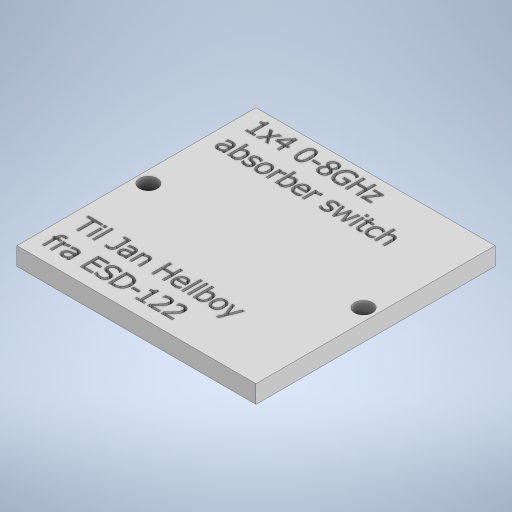
# Autodesk Inventor part: switch cover
Saved by Autodesk Inventor 2023.5 (Build 275446000, 446)
## iProperties
Created: 2025-10-22
Part Number: switch cover
Material: Generic
Document SubType Name: Modeling
Designer: Mikke
Density: 1 g/cm^3
Appearance: Default
Author: Mikke
Autodesk Inventor part; units mm, degrees
(part 1 of 2)
ref_plane "YZ Plane" through (0, 0, 0) normal (1, 0, 0) x (0, 1, 0)
ref_plane "XZ Plane" through (0, 0, 0) normal (0, 1, 0) x (-1, 0, 0)
ref_plane "XY Plane" through (0, 0, 0) normal (0, 0, 1) x (1, 0, 0)
sketch "Sketch1" plane through (0, 0, 0) normal (0, 1, 0) x (-1, 0, 0)
  line L0 (-20, 20) -> (20, 20)
  line L1 (20, 20) -> (20, -20)
  line L2 (20, -20) -> (-20, -20)
  line L3 (-20, -20) -> (-20, 20)
  line L4 (-20, 20) -> (20, -20) construction
  line L5 (20, 20) -> (-20, -20) construction
  line L6 (20, 0) -> (18, 0)
  circle A0 centre (18, 0) radius 1.5
  line L7 (-20, 0) -> (-18, 0)
  circle A1 centre (-18, 0) radius 1.5
  point P0 (0, 0)
  dimension "d0" = 40
  dimension "d1" = 40
  dimension "d2" = 2
  dimension "d3" = 3
  dimension "d4" = 2
  dimension "d5" = 3
  constraints: 16 end point, 4 midpoint, 3 horizontal, 2 centre point, 2 coincident, 2 parallel, 1 perpendicular
  measures "d0" distance of L1.end L2.end
  measures "d1" distance of L0.end L1.end
  measures "d2" distance of L6.start L6.end
  measures "d3" diameter of A0
  measures "d4" distance of L7.start L7.end
  measures "d5" diameter of A1
extrude "Extrusion1" add sketch "Sketch1" along normal blind 3
sketch "Sketch2" plane through (0, 3, 0) normal (0, 1, 0) x (1, 0, 0)
  line L0 (-18.035, 18.8782) -> (18.3992, 18.8782) construction
  line L1 (18.3992, 18.8782) -> (18.3992, 9.0682) construction
  line L2 (18.3992, 9.0682) -> (-18.035, 9.0682) construction
  line L3 (-18.035, 9.0682) -> (-18.035, 18.8782) construction
  line L4 (-18.3377, -9.5579) -> (18.7673, -9.5579) construction
  line L5 (18.7673, -9.5579) -> (18.7673, -19.1286) construction
  line L6 (18.7673, -19.1286) -> (-18.3377, -19.1286) construction
  line L7 (-18.3377, -19.1286) -> (-18.3377, -9.5579) construction
  line L8 (-16.0862, 15.761) -> (-17.5731, 15.761)
  line L9 (-17.5731, 15.761) -> (-17.5731, 16.0722)
  line L10 (-17.5731, 16.0722) -> (-17.0198, 16.0722)
  line L11 (-17.0198, 16.0722) -> (-17.0198, 18.1149)
  line L12 (-17.0198, 18.1149) -> (-17.5731, 18.1149)
  line L13 (-17.5731, 18.1149) -> (-17.5731, 18.394)
  spline S0 degree 2 poles (-17.5731, 18.394) (-17.2594, 18.394) (-16.963, 18.5719) (-16.9433, 18.8189) knots 0 0 0 1 2 2 2
  line L14 (-16.9433, 18.8189) -> (-16.6271, 18.8189)
  line L15 (-16.6271, 18.8189) -> (-16.6271, 16.0722)
  line L16 (-16.6271, 16.0722) -> (-16.0862, 16.0722)
  line L17 (-16.0862, 16.0722) -> (-16.0862, 15.761)
  line L18 (-13.6927, 15.761) -> (-14.1645, 15.761)
  line L19 (-14.1645, 15.761) -> (-14.7203, 16.6206)
  line L20 (-14.7203, 16.6206) -> (-15.2908, 15.761)
  line L21 (-15.2908, 15.761) -> (-15.728, 15.761)
  line L22 (-15.728, 15.761) -> (-14.9352, 16.8947)
  line L23 (-14.9352, 16.8947) -> (-15.7206, 18.0482)
  line L24 (-15.7206, 18.0482) -> (-15.2488, 18.0482)
  line L25 (-15.2488, 18.0482) -> (-14.6956, 17.1961)
  line L26 (-14.6956, 17.1961) -> (-14.1299, 18.0482)
  line L27 (-14.1299, 18.0482) -> (-13.6927, 18.0482)
  line L28 (-13.6927, 18.0482) -> (-14.4807, 16.9194)
  line L29 (-14.4807, 16.9194) -> (-13.6927, 15.761)
  line L30 (-11.4895, 16.8083) -> (-11.8526, 16.8083)
  line L31 (-11.8526, 16.8083) -> (-11.8526, 15.761)
  line L32 (-11.8526, 15.761) -> (-12.2453, 15.761)
  line L33 (-12.2453, 15.761) -> (-12.2453, 16.8083)
  line L34 (-12.2453, 16.8083) -> (-13.5915, 16.8083)
  line L35 (-13.5915, 16.8083) -> (-13.5915, 17.2381)
  line L36 (-13.5915, 17.2381) -> (-12.228, 18.809)
  line L37 (-12.228, 18.809) -> (-11.8526, 18.809)
  line L38 (-11.8526, 18.809) -> (-11.8526, 17.1368)
  line L39 (-11.8526, 17.1368) -> (-11.4895, 17.1368)
  line L40 (-11.4895, 17.1368) -> (-11.4895, 16.8083)
  line L41 (-12.2453, 17.1368) -> (-12.2453, 18.3274)
  line L42 (-12.2453, 18.3274) -> (-13.2704, 17.1368)
  line L43 (-13.2704, 17.1368) -> (-12.2453, 17.1368)
  spline S1 degree 2 poles (-7.9574, 17.285) (-7.9574, 16.465) (-8.4341, 15.6968) (-8.9305, 15.6968) knots 0 0 0 1 2 2 2
  spline S2 degree 2 poles (-8.9305, 15.6968) (-9.4344, 15.6968) (-9.9062, 16.4798) (-9.9062, 17.2825) knots 0 0 0 1 2 2 2
  spline S3 degree 2 poles (-9.9062, 17.2825) (-9.9062, 18.1075) (-9.4295, 18.8708) (-8.9305, 18.8708) knots 0 0 0 1 2 2 2
  spline S4 degree 2 poles (-8.9305, 18.8708) (-8.4291, 18.8708) (-7.9574, 18.0804) (-7.9574, 17.285) knots 0 0 0 1 2 2 2
  spline S5 degree 2 poles (-8.481, 16.3563) (-8.4217, 16.507) (-8.3723, 16.9713) (-8.3723, 17.285) knots 0 0 0 1 2 2 2
  spline S6 degree 2 poles (-8.3723, 17.285) (-8.3723, 17.5987) (-8.4217, 18.0606) (-8.4835, 18.2162) knots 0 0 0 1 2 2 2
  spline S7 degree 2 poles (-8.4835, 18.2162) (-8.5452, 18.3718) (-8.7601, 18.5324) (-8.9305, 18.5324) knots 0 0 0 1 2 2 2
  spline S8 degree 2 poles (-8.9305, 18.5324) (-9.101, 18.5324) (-9.3208, 18.3718) (-9.385, 18.2113) knots 0 0 0 1 2 2 2
  spline S9 degree 2 poles (-9.385, 18.2113) (-9.4468, 18.0557) (-9.4912, 17.5814) (-9.4912, 17.2825) knots 0 0 0 1 2 2 2
  spline S10 degree 2 poles (-9.4912, 17.2825) (-9.4912, 16.9614) (-9.4517, 16.5317) (-9.3875, 16.3637) knots 0 0 0 1 2 2 2
  spline S11 degree 2 poles (-9.3875, 16.3637) (-9.3282, 16.2056) (-9.1084, 16.0352) (-8.9305, 16.0352) knots 0 0 0 1 2 2 2
  spline S12 degree 2 poles (-8.9305, 16.0352) (-8.7626, 16.0352) (-8.5428, 16.1957) (-8.481, 16.3563) knots 0 0 0 1 2 2 2
  line L44 (-6.4506, 16.9096) -> (-7.6041, 16.9096)
  line L45 (-7.6041, 16.9096) -> (-7.6041, 17.2801)
  line L46 (-7.6041, 17.2801) -> (-6.4506, 17.2801)
  line L47 (-6.4506, 17.2801) -> (-6.4506, 16.9096)
  spline S13 degree 2 poles (-5.1243, 15.6918) (-5.3515, 15.6918) (-5.7245, 15.8277) (-5.8554, 15.9537) knots 0 0 0 1 2 2 2
  spline S14 degree 2 poles (-5.8554, 15.9537) (-5.9838, 16.0772) (-6.1172, 16.4131) (-6.1172, 16.6033) knots 0 0 0 1 2 2 2
  spline S15 degree 2 poles (-6.1172, 16.6033) (-6.1172, 16.8503) (-5.8529, 17.2652) (-5.601, 17.3887) knots 0 0 0 1 2 2 2
  line L48 (-5.601, 17.3887) -> (-5.601, 17.4011)
  spline S16 degree 2 poles (-5.601, 17.4011) (-5.8257, 17.532) (-6.0431, 17.8432) (-6.0431, 18.0754) knots 0 0 0 1 2 2 2
  spline S17 degree 2 poles (-6.0431, 18.0754) (-6.0431, 18.4187) (-5.5244, 18.8782) (-5.1243, 18.8782) knots 0 0 0 1 2 2 2
  spline S18 degree 2 poles (-5.1243, 18.8782) (-4.7093, 18.8782) (-4.2079, 18.4434) (-4.2079, 18.1026) knots 0 0 0 1 2 2 2
  spline S19 degree 2 poles (-4.2079, 18.1026) (-4.2079, 17.8976) (-4.4475, 17.4974) (-4.6722, 17.3838) knots 0 0 0 1 2 2 2
  line L49 (-4.6722, 17.3838) -> (-4.6722, 17.3715)
  spline S20 degree 2 poles (-4.6722, 17.3715) (-4.4055, 17.248) (-4.1313, 16.8923) (-4.1313, 16.6107) knots 0 0 0 1 2 2 2
  spline S21 degree 2 poles (-4.1313, 16.6107) (-4.1313, 16.2204) (-4.6994, 15.6918) (-5.1243, 15.6918) knots 0 0 0 1 2 2 2
  spline S22 degree 2 poles (-4.5512, 16.5712) (-4.5512, 16.7589) (-4.6994, 16.9812) (-4.9094, 17.0948) knots 0 0 0 1 2 2 2
  spline S23 degree 2 poles (-4.9094, 17.0948) (-4.9785, 17.1343) (-5.2107, 17.2257) (-5.3564, 17.285) knots 0 0 0 1 2 2 2
  spline S24 degree 2 poles (-5.3564, 17.285) (-5.5244, 17.1739) (-5.7047, 16.8429) (-5.7047, 16.6329) knots 0 0 0 1 2 2 2
  spline S25 degree 2 poles (-5.7047, 16.6329) (-5.7047, 16.3563) (-5.3713, 15.9957) (-5.1193, 15.9957) knots 0 0 0 1 2 2 2
  spline S26 degree 2 poles (-5.1193, 15.9957) (-4.8624, 15.9957) (-4.5512, 16.3044) (-4.5512, 16.5712) knots 0 0 0 1 2 2 2
  spline S27 degree 2 poles (-4.608, 18.0976) (-4.608, 18.3027) (-4.8822, 18.5768) (-5.1267, 18.5768) knots 0 0 0 1 2 2 2
  spline S28 degree 2 poles (-5.1267, 18.5768) (-5.349, 18.5768) (-5.6331, 18.3323) (-5.6331, 18.1223) knots 0 0 0 1 2 2 2
  spline S29 degree 2 poles (-5.6331, 18.1223) (-5.6331, 17.9717) (-5.4873, 17.7617) (-5.3416, 17.6777) knots 0 0 0 1 2 2 2
  spline S30 degree 2 poles (-5.3416, 17.6777) (-5.2799, 17.6432) (-5.018, 17.5221) (-4.9118, 17.4875) knots 0 0 0 1 2 2 2
  spline S31 degree 2 poles (-4.9118, 17.4875) (-4.734, 17.6234) (-4.608, 17.9124) (-4.608, 18.0976) knots 0 0 0 1 2 2 2
  spline S32 degree 2 poles (-2.3949, 15.7017) (-2.7185, 15.7017) (-3.2544, 15.8993) (-3.4471, 16.0994) knots 0 0 0 1 2 2 2
  spline S33 degree 2 poles (-3.4471, 16.0994) (-3.6398, 16.3019) (-3.8448, 16.8997) (-3.8448, 17.2875) knots 0 0 0 1 2 2 2
  spline S34 degree 2 poles (-3.8448, 17.2875) (-3.8448, 17.6555) (-3.6373, 18.2384) (-3.4446, 18.4459) knots 0 0 0 1 2 2 2
  spline S35 degree 2 poles (-3.4446, 18.4459) (-3.2594, 18.646) (-2.716, 18.8633) (-2.3924, 18.8633) knots 0 0 0 1 2 2 2
  spline S36 degree 2 poles (-2.3924, 18.8633) (-2.2368, 18.8633) (-1.9552, 18.8189) (-1.8268, 18.7794) knots 0 0 0 1 2 2 2
  spline S37 degree 2 poles (-1.8268, 18.7794) (-1.723, 18.7497) (-1.4711, 18.641) (-1.3945, 18.6015) knots 0 0 0 1 2 2 2
  line L50 (-1.3945, 18.6015) -> (-1.3945, 18.1125)
  line L51 (-1.3945, 18.1125) -> (-1.4291, 18.1125)
  spline S38 degree 2 poles (-1.4291, 18.1125) (-1.5057, 18.1792) (-1.6662, 18.3002) (-1.8144, 18.3693) knots 0 0 0 1 2 2 2
  spline S39 degree 2 poles (-1.8144, 18.3693) (-1.9379, 18.4311) (-2.2566, 18.5126) (-2.4393, 18.5126) knots 0 0 0 1 2 2 2
  spline S40 degree 2 poles (-2.4393, 18.5126) (-2.879, 18.5126) (-3.4224, 17.8506) (-3.4224, 17.2998) knots 0 0 0 1 2 2 2
  spline S41 degree 2 poles (-3.4224, 17.2998) (-3.4224, 16.9935) (-3.2791, 16.5341) (-3.1433, 16.376) knots 0 0 0 1 2 2 2
  spline S42 degree 2 poles (-3.1433, 16.376) (-3.0124, 16.218) (-2.6419, 16.0525) (-2.4097, 16.0525) knots 0 0 0 1 2 2 2
  spline S43 degree 2 poles (-2.4097, 16.0525) (-2.2393, 16.0525) (-1.8984, 16.1019) (-1.7823, 16.1513) knots 0 0 0 1 2 2 2
  line L52 (-1.7823, 16.1513) -> (-1.7823, 16.9392)
  line L53 (-1.7823, 16.9392) -> (-2.4887, 16.9392)
  line L54 (-2.4887, 16.9392) -> (-2.4887, 17.2949)
  line L55 (-2.4887, 17.2949) -> (-1.3822, 17.2949)
  line L56 (-1.3822, 17.2949) -> (-1.3822, 15.9635)
  spline S44 degree 2 poles (-1.3822, 15.9635) (-1.4587, 15.929) (-1.7206, 15.8228) (-1.8317, 15.7906) knots 0 0 0 1 2 2 2
  spline S45 degree 2 poles (-1.8317, 15.7906) (-1.9824, 15.7462) (-2.2245, 15.7017) (-2.3949, 15.7017) knots 0 0 0 1 2 2 2
  line L57 (1.3398, 15.761) -> (0.9347, 15.761)
  line L58 (0.9347, 15.761) -> (0.9347, 17.2529)
  line L59 (0.9347, 17.2529) -> (-0.4683, 17.2529)
  line L60 (-0.4683, 17.2529) -> (-0.4683, 15.761)
  line L61 (-0.4683, 15.761) -> (-0.8734, 15.761)
  line L62 (-0.8734, 15.761) -> (-0.8734, 18.809)
  line L63 (-0.8734, 18.809) -> (-0.4683, 18.809)
  line L64 (-0.4683, 18.809) -> (-0.4683, 17.6135)
  line L65 (-0.4683, 17.6135) -> (0.9347, 17.6135)
  line L66 (0.9347, 17.6135) -> (0.9347, 18.809)
  line L67 (0.9347, 18.809) -> (1.3398, 18.809)
  line L68 (1.3398, 18.809) -> (1.3398, 15.761)
  line L69 (3.4294, 15.761) -> (1.7498, 15.761)
  line L70 (1.7498, 15.761) -> (1.7498, 16.0475)
  line L71 (1.7498, 16.0475) -> (2.9453, 17.7321)
  line L72 (2.9453, 17.7321) -> (1.7992, 17.7321)
  line L73 (1.7992, 17.7321) -> (1.7992, 18.0482)
  line L74 (1.7992, 18.0482) -> (3.4072, 18.0482)
  line L75 (3.4072, 18.0482) -> (3.4072, 17.7741)
  line L76 (3.4072, 17.7741) -> (2.2068, 16.0846)
  line L77 (2.2068, 16.0846) -> (3.4294, 16.0846)
  line L78 (3.4294, 16.0846) -> (3.4294, 15.761)
  spline S46 degree 2 poles (-16.4814, 10.9846) (-16.5283, 10.95) (-16.6864, 10.8265) (-16.7605, 10.7895) knots 0 0 0 1 2 2 2
  spline S47 degree 2 poles (-16.7605, 10.7895) (-16.8618, 10.7351) (-17.052, 10.6783) (-17.2249, 10.6783) knots 0 0 0 1 2 2 2
  spline S48 degree 2 poles (-17.2249, 10.6783) (-17.3657, 10.6783) (-17.6201, 10.7845) (-17.7164, 10.8809) knots 0 0 0 1 2 2 2
  spline S49 degree 2 poles (-17.7164, 10.8809) (-17.8078, 10.9747) (-17.9189, 11.2514) (-17.9189, 11.4045) knots 0 0 0 1 2 2 2
  spline S50 degree 2 poles (-17.9189, 11.4045) (-17.9189, 11.6416) (-17.7189, 11.9776) (-17.5015, 12.0739) knots 0 0 0 1 2 2 2
  spline S51 degree 2 poles (-17.5015, 12.0739) (-17.3088, 12.1628) (-16.7852, 12.2295) (-16.4814, 12.2468) knots 0 0 0 1 2 2 2
  line L79 (-16.4814, 12.2468) -> (-16.4814, 12.3209)
  spline S52 degree 2 poles (-16.4814, 12.3209) (-16.4814, 12.4543) (-16.5629, 12.6198) (-16.637, 12.6667) knots 0 0 0 1 2 2 2
  spline S53 degree 2 poles (-16.637, 12.6667) (-16.7111, 12.7136) (-16.9235, 12.7433) (-17.0371, 12.7433) knots 0 0 0 1 2 2 2
  spline S54 degree 2 poles (-17.0371, 12.7433) (-17.1705, 12.7433) (-17.5311, 12.6642) (-17.7115, 12.5877) knots 0 0 0 1 2 2 2
  line L80 (-17.7115, 12.5877) -> (-17.7337, 12.5877)
  line L81 (-17.7337, 12.5877) -> (-17.7337, 12.9804)
  spline S55 degree 2 poles (-17.7337, 12.9804) (-17.6275, 13.01) (-17.2298, 13.0841) (-17.0347, 13.0841) knots 0 0 0 1 2 2 2
  spline S56 degree 2 poles (-17.0347, 13.0841) (-16.7975, 13.0841) (-16.474, 13.01) (-16.3455, 12.9137) knots 0 0 0 1 2 2 2
  spline S57 degree 2 poles (-16.3455, 12.9137) (-16.2196, 12.8198) (-16.0961, 12.521) (-16.0961, 12.3061) knots 0 0 0 1 2 2 2
  line L82 (-16.0961, 12.3061) -> (-16.0961, 10.7426)
  line L83 (-16.0961, 10.7426) -> (-16.4814, 10.7426)
  line L84 (-16.4814, 10.7426) -> (-16.4814, 10.9846)
  line L85 (-16.4814, 11.3057) -> (-16.4814, 11.9405)
  spline S58 degree 2 poles (-16.4814, 11.9405) (-16.6197, 11.9282) (-17.0371, 11.8862) (-17.168, 11.8467) knots 0 0 0 1 2 2 2
  spline S59 degree 2 poles (-17.168, 11.8467) (-17.3212, 11.7997) (-17.5213, 11.6046) (-17.5213, 11.4317) knots 0 0 0 1 2 2 2
  spline S60 degree 2 poles (-17.5213, 11.4317) (-17.5213, 11.2341) (-17.299, 11.034) (-17.0865, 11.034) knots 0 0 0 1 2 2 2
  spline S61 degree 2 poles (-17.0865, 11.034) (-16.9062, 11.034) (-16.6098, 11.1896) (-16.4814, 11.3057) knots 0 0 0 1 2 2 2
  spline S62 degree 2 poles (-13.6384, 11.9232) (-13.6384, 11.3625) (-14.1818, 10.6783) (-14.5918, 10.6783) knots 0 0 0 1 2 2 2
  spline S63 degree 2 poles (-14.5918, 10.6783) (-14.7771, 10.6783) (-15.0414, 10.7697) (-15.1698, 10.8488) knots 0 0 0 1 2 2 2
  line L86 (-15.1698, 10.8488) -> (-15.1945, 10.7426)
  line L87 (-15.1945, 10.7426) -> (-15.5551, 10.7426)
  line L88 (-15.5551, 10.7426) -> (-15.5551, 13.9264)
  line L89 (-15.5551, 13.9264) -> (-15.1698, 13.9264)
  line L90 (-15.1698, 13.9264) -> (-15.1698, 12.7902)
  spline S64 degree 2 poles (-15.1698, 12.7902) (-15.0241, 12.9211) (-14.6857, 13.094) (-14.4708, 13.094) knots 0 0 0 1 2 2 2
  spline S65 degree 2 poles (-14.4708, 13.094) (-14.083, 13.094) (-13.6384, 12.474) (-13.6384, 11.9232) knots 0 0 0 1 2 2 2
  spline S66 degree 2 poles (-14.0361, 11.8936) (-14.0361, 12.3036) (-14.2855, 12.7284) (-14.5622, 12.7284) knots 0 0 0 1 2 2 2
  spline S67 degree 2 poles (-14.5622, 12.7284) (-14.7178, 12.7284) (-15.0389, 12.5802) (-15.1698, 12.4666) knots 0 0 0 1 2 2 2
  line L91 (-15.1698, 12.4666) -> (-15.1698, 11.155)
  spline S68 degree 2 poles (-15.1698, 11.155) (-15.0241, 11.0834) (-14.7993, 11.0241) (-14.6659, 11.0241) knots 0 0 0 1 2 2 2
  spline S69 degree 2 poles (-14.6659, 11.0241) (-14.372, 11.0241) (-14.0361, 11.4416) (-14.0361, 11.8936) knots 0 0 0 1 2 2 2
  spline S70 degree 2 poles (-12.6207, 10.6882) (-12.8505, 10.6882) (-13.2481, 10.8117) (-13.379, 10.8809) knots 0 0 0 1 2 2 2
  line L92 (-13.379, 10.8809) -> (-13.379, 11.3131)
  line L93 (-13.379, 11.3131) -> (-13.3593, 11.3131)
  spline S71 degree 2 poles (-13.3593, 11.3131) (-13.3099, 11.2736) (-13.1765, 11.1797) (-13.0654, 11.1279) knots 0 0 0 1 2 2 2
  spline S72 degree 2 poles (-13.0654, 11.1279) (-12.969, 11.0809) (-12.7319, 11.0118) (-12.6059, 11.0118) knots 0 0 0 1 2 2 2
  spline S73 degree 2 poles (-12.6059, 11.0118) (-12.5145, 11.0118) (-12.3046, 11.0538) (-12.2552, 11.0884) knots 0 0 0 1 2 2 2
  spline S74 degree 2 poles (-12.2552, 11.0884) (-12.1836, 11.1353) (-12.1193, 11.2415) (-12.1193, 11.3502) knots 0 0 0 1 2 2 2
  spline S75 degree 2 poles (-12.1193, 11.3502) (-12.1193, 11.486) (-12.2675, 11.6268) (-12.4577, 11.6738) knots 0 0 0 1 2 2 2
  spline S76 degree 2 poles (-12.4577, 11.6738) (-12.5318, 11.691) (-12.769, 11.7404) (-12.8702, 11.7676) knots 0 0 0 1 2 2 2
  spline S77 degree 2 poles (-12.8702, 11.7676) (-13.132, 11.8442) (-13.3692, 12.1603) (-13.3692, 12.3851) knots 0 0 0 1 2 2 2
  spline S78 degree 2 poles (-13.3692, 12.3851) (-13.3692, 12.6963) (-12.9023, 13.0841) (-12.517, 13.0841) knots 0 0 0 1 2 2 2
  spline S79 degree 2 poles (-12.517, 13.0841) (-12.3268, 13.0841) (-11.9415, 12.9903) (-11.8106, 12.9186) knots 0 0 0 1 2 2 2
  line L94 (-11.8106, 12.9186) -> (-11.8106, 12.5061)
  line L95 (-11.8106, 12.5061) -> (-11.8303, 12.5061)
  spline S80 degree 2 poles (-11.8303, 12.5061) (-11.9785, 12.6247) (-12.3392, 12.7606) (-12.5244, 12.7606) knots 0 0 0 1 2 2 2
  spline S81 degree 2 poles (-12.5244, 12.7606) (-12.7146, 12.7606) (-12.9764, 12.6) (-12.9764, 12.4395) knots 0 0 0 1 2 2 2
  spline S82 degree 2 poles (-12.9764, 12.4395) (-12.9764, 12.2937) (-12.8208, 12.1529) (-12.6479, 12.1085) knots 0 0 0 1 2 2 2
  spline S83 degree 2 poles (-12.6479, 12.1085) (-12.5639, 12.0862) (-12.3515, 12.0418) (-12.2354, 12.0146) knots 0 0 0 1 2 2 2
  spline S84 degree 2 poles (-12.2354, 12.0146) (-11.9835, 11.9504) (-11.7266, 11.6565) (-11.7266, 11.402) knots 0 0 0 1 2 2 2
  spline S85 degree 2 poles (-11.7266, 11.402) (-11.7266, 11.2538) (-11.8427, 10.992) (-11.9563, 10.8957) knots 0 0 0 1 2 2 2
  spline S86 degree 2 poles (-11.9563, 10.8957) (-12.0773, 10.7944) (-12.3861, 10.6882) (-12.6207, 10.6882) knots 0 0 0 1 2 2 2
  spline S87 degree 2 poles (-9.4888, 11.8862) (-9.4888, 11.3082) (-10.0445, 10.6783) (-10.5089, 10.6783) knots 0 0 0 1 2 2 2
  spline S88 degree 2 poles (-10.5089, 10.6783) (-10.9856, 10.6783) (-11.5315, 11.3279) (-11.5315, 11.8862) knots 0 0 0 1 2 2 2
  spline S89 degree 2 poles (-11.5315, 11.8862) (-11.5315, 12.4592) (-10.9683, 13.094) (-10.5089, 13.094) knots 0 0 0 1 2 2 2
  spline S90 degree 2 poles (-10.5089, 13.094) (-10.0445, 13.094) (-9.4888, 12.4617) (-9.4888, 11.8862) knots 0 0 0 1 2 2 2
  spline S91 degree 2 poles (-9.8864, 11.8862) (-9.8864, 12.3308) (-10.21, 12.763) (-10.5089, 12.763) knots 0 0 0 1 2 2 2
  spline S92 degree 2 poles (-10.5089, 12.763) (-10.8078, 12.763) (-11.1338, 12.3308) (-11.1338, 11.8862) knots 0 0 0 1 2 2 2
  spline S93 degree 2 poles (-11.1338, 11.8862) (-11.1338, 11.4539) (-10.8078, 11.0093) (-10.5089, 11.0093) knots 0 0 0 1 2 2 2
  spline S94 degree 2 poles (-10.5089, 11.0093) (-10.2125, 11.0093) (-9.8864, 11.4465) (-9.8864, 11.8862) knots 0 0 0 1 2 2 2
  line L96 (-7.8808, 12.6173) -> (-7.9005, 12.6173)
  spline S95 degree 2 poles (-7.9005, 12.6173) (-7.945, 12.6296) (-8.0413, 12.6346) (-8.108, 12.6346) knots 0 0 0 1 2 2 2
  spline S96 degree 2 poles (-8.108, 12.6346) (-8.2636, 12.6346) (-8.5699, 12.4987) (-8.7082, 12.3654) knots 0 0 0 1 2 2 2
  line L97 (-8.7082, 12.3654) -> (-8.7082, 10.7426)
  line L98 (-8.7082, 10.7426) -> (-9.0936, 10.7426)
  line L99 (-9.0936, 10.7426) -> (-9.0936, 13.0298)
  line L100 (-9.0936, 13.0298) -> (-8.7082, 13.0298)
  line L101 (-8.7082, 13.0298) -> (-8.7082, 12.6889)
  spline S97 degree 2 poles (-8.7082, 12.6889) (-8.4983, 12.8766) (-8.1846, 13.0298) (-8.0364, 13.0298) knots 0 0 0 1 2 2 2
  spline S98 degree 2 poles (-8.0364, 13.0298) (-7.9771, 13.0298) (-7.9178, 13.0248) (-7.8808, 13.0174) knots 0 0 0 1 2 2 2
  line L102 (-7.8808, 13.0174) -> (-7.8808, 12.6173)
  spline S99 degree 2 poles (-5.6652, 11.9232) (-5.6652, 11.3625) (-6.2086, 10.6783) (-6.6186, 10.6783) knots 0 0 0 1 2 2 2
  spline S100 degree 2 poles (-6.6186, 10.6783) (-6.8039, 10.6783) (-7.0682, 10.7697) (-7.1966, 10.8488) knots 0 0 0 1 2 2 2
  line L103 (-7.1966, 10.8488) -> (-7.2213, 10.7426)
  line L104 (-7.2213, 10.7426) -> (-7.5819, 10.7426)
  line L105 (-7.5819, 10.7426) -> (-7.5819, 13.9264)
  line L106 (-7.5819, 13.9264) -> (-7.1966, 13.9264)
  line L107 (-7.1966, 13.9264) -> (-7.1966, 12.7902)
  spline S101 degree 2 poles (-7.1966, 12.7902) (-7.0509, 12.9211) (-6.7125, 13.094) (-6.4976, 13.094) knots 0 0 0 1 2 2 2
  spline S102 degree 2 poles (-6.4976, 13.094) (-6.1098, 13.094) (-5.6652, 12.474) (-5.6652, 11.9232) knots 0 0 0 1 2 2 2
  spline S103 degree 2 poles (-6.0629, 11.8936) (-6.0629, 12.3036) (-6.3123, 12.7284) (-6.589, 12.7284) knots 0 0 0 1 2 2 2
  spline S104 degree 2 poles (-6.589, 12.7284) (-6.7446, 12.7284) (-7.0657, 12.5802) (-7.1966, 12.4666) knots 0 0 0 1 2 2 2
  line L108 (-7.1966, 12.4666) -> (-7.1966, 11.155)
  spline S105 degree 2 poles (-7.1966, 11.155) (-7.0509, 11.0834) (-6.8261, 11.0241) (-6.6927, 11.0241) knots 0 0 0 1 2 2 2
  spline S106 degree 2 poles (-6.6927, 11.0241) (-6.3988, 11.0241) (-6.0629, 11.4416) (-6.0629, 11.8936) knots 0 0 0 1 2 2 2
  spline S107 degree 2 poles (-4.2721, 10.6907) (-4.8204, 10.6907) (-5.4231, 11.3057) (-5.4231, 11.8738) knots 0 0 0 1 2 2 2
  spline S108 degree 2 poles (-5.4231, 11.8738) (-5.4231, 12.432) (-4.8377, 13.094) (-4.366, 13.094) knots 0 0 0 1 2 2 2
  spline S109 degree 2 poles (-4.366, 13.094) (-4.1535, 13.094) (-3.825, 12.9705) (-3.704, 12.8396) knots 0 0 0 1 2 2 2
  spline S110 degree 2 poles (-3.704, 12.8396) (-3.5805, 12.7087) (-3.4496, 12.3308) (-3.4496, 12.0566) knots 0 0 0 1 2 2 2
  line L109 (-3.4496, 12.0566) -> (-3.4496, 11.8467)
  line L110 (-3.4496, 11.8467) -> (-5.0329, 11.8467)
  spline S111 degree 2 poles (-5.0329, 11.8467) (-5.0329, 11.449) (-4.6327, 11.0266) (-4.277, 11.0266) knots 0 0 0 1 2 2 2
  spline S112 degree 2 poles (-4.277, 11.0266) (-4.1511, 11.0266) (-3.9065, 11.0834) (-3.8077, 11.1279) knots 0 0 0 1 2 2 2
  spline S113 degree 2 poles (-3.8077, 11.1279) (-3.704, 11.1773) (-3.5607, 11.2637) (-3.5138, 11.3032) knots 0 0 0 1 2 2 2
  line L111 (-3.5138, 11.3032) -> (-3.4916, 11.3032)
  line L112 (-3.4916, 11.3032) -> (-3.4916, 10.8833)
  spline S114 degree 2 poles (-3.4916, 10.8833) (-3.5583, 10.8562) (-3.7608, 10.7771) (-3.8398, 10.7549) knots 0 0 0 1 2 2 2
  spline S115 degree 2 poles (-3.8398, 10.7549) (-3.951, 10.7228) (-4.1338, 10.6907) (-4.2721, 10.6907) knots 0 0 0 1 2 2 2
  spline S116 degree 2 poles (-3.825, 12.1406) (-3.83, 12.2962) (-3.8942, 12.5234) (-3.9559, 12.6) knots 0 0 0 1 2 2 2
  spline S117 degree 2 poles (-3.9559, 12.6) (-4.0226, 12.6865) (-4.2326, 12.7778) (-4.3882, 12.7778) knots 0 0 0 1 2 2 2
  spline S118 degree 2 poles (-4.3882, 12.7778) (-4.5413, 12.7778) (-4.7562, 12.6865) (-4.8451, 12.5975) knots 0 0 0 1 2 2 2
  spline S119 degree 2 poles (-4.8451, 12.5975) (-4.9316, 12.5061) (-5.0205, 12.2863) (-5.0329, 12.1406) knots 0 0 0 1 2 2 2
  line L113 (-5.0329, 12.1406) -> (-3.825, 12.1406)
  line L114 (-1.8465, 12.6173) -> (-1.8663, 12.6173)
  spline S120 degree 2 poles (-1.8663, 12.6173) (-1.9108, 12.6296) (-2.0071, 12.6346) (-2.0738, 12.6346) knots 0 0 0 1 2 2 2
  spline S121 degree 2 poles (-2.0738, 12.6346) (-2.2294, 12.6346) (-2.5357, 12.4987) (-2.674, 12.3654) knots 0 0 0 1 2 2 2
  line L115 (-2.674, 12.3654) -> (-2.674, 10.7426)
  line L116 (-2.674, 10.7426) -> (-3.0593, 10.7426)
  line L117 (-3.0593, 10.7426) -> (-3.0593, 13.0298)
  line L118 (-3.0593, 13.0298) -> (-2.674, 13.0298)
  line L119 (-2.674, 13.0298) -> (-2.674, 12.6889)
  spline S122 degree 2 poles (-2.674, 12.6889) (-2.464, 12.8766) (-2.1504, 13.0298) (-2.0021, 13.0298) knots 0 0 0 1 2 2 2
  spline S123 degree 2 poles (-2.0021, 13.0298) (-1.9429, 13.0298) (-1.8836, 13.0248) (-1.8465, 13.0174) knots 0 0 0 1 2 2 2
  line L120 (-1.8465, 13.0174) -> (-1.8465, 12.6173)
  spline S124 degree 2 poles (0.3789, 10.6882) (0.1492, 10.6882) (-0.2484, 10.8117) (-0.3793, 10.8809) knots 0 0 0 1 2 2 2
  line L121 (-0.3793, 10.8809) -> (-0.3793, 11.3131)
  line L122 (-0.3793, 11.3131) -> (-0.3596, 11.3131)
  spline S125 degree 2 poles (-0.3596, 11.3131) (-0.3102, 11.2736) (-0.1768, 11.1797) (-0.0657, 11.1279) knots 0 0 0 1 2 2 2
  spline S126 degree 2 poles (-0.0657, 11.1279) (0.0307, 11.0809) (0.2678, 11.0118) (0.3938, 11.0118) knots 0 0 0 1 2 2 2
  spline S127 degree 2 poles (0.3938, 11.0118) (0.4852, 11.0118) (0.6951, 11.0538) (0.7445, 11.0884) knots 0 0 0 1 2 2 2
  spline S128 degree 2 poles (0.7445, 11.0884) (0.8161, 11.1353) (0.8804, 11.2415) (0.8804, 11.3502) knots 0 0 0 1 2 2 2
  spline S129 degree 2 poles (0.8804, 11.3502) (0.8804, 11.486) (0.7322, 11.6268) (0.542, 11.6738) knots 0 0 0 1 2 2 2
  spline S130 degree 2 poles (0.542, 11.6738) (0.4679, 11.691) (0.2307, 11.7404) (0.1295, 11.7676) knots 0 0 0 1 2 2 2
  spline S131 degree 2 poles (0.1295, 11.7676) (-0.1323, 11.8442) (-0.3695, 12.1603) (-0.3695, 12.3851) knots 0 0 0 1 2 2 2
  spline S132 degree 2 poles (-0.3695, 12.3851) (-0.3695, 12.6963) (0.0974, 13.0841) (0.4827, 13.0841) knots 0 0 0 1 2 2 2
  spline S133 degree 2 poles (0.4827, 13.0841) (0.6729, 13.0841) (1.0582, 12.9903) (1.1891, 12.9186) knots 0 0 0 1 2 2 2
  line L123 (1.1891, 12.9186) -> (1.1891, 12.5061)
  line L124 (1.1891, 12.5061) -> (1.1694, 12.5061)
  spline S134 degree 2 poles (1.1694, 12.5061) (1.0212, 12.6247) (0.6605, 12.7606) (0.4753, 12.7606) knots 0 0 0 1 2 2 2
  spline S135 degree 2 poles (0.4753, 12.7606) (0.2851, 12.7606) (0.0233, 12.6) (0.0233, 12.4395) knots 0 0 0 1 2 2 2
  spline S136 degree 2 poles (0.0233, 12.4395) (0.0233, 12.2937) (0.1789, 12.1529) (0.3518, 12.1085) knots 0 0 0 1 2 2 2
  spline S137 degree 2 poles (0.3518, 12.1085) (0.4358, 12.0862) (0.6482, 12.0418) (0.7643, 12.0146) knots 0 0 0 1 2 2 2
  spline S138 degree 2 poles (0.7643, 12.0146) (1.0162, 11.9504) (1.2731, 11.6565) (1.2731, 11.402) knots 0 0 0 1 2 2 2
  spline S139 degree 2 poles (1.2731, 11.402) (1.2731, 11.2538) (1.157, 10.992) (1.0434, 10.8957) knots 0 0 0 1 2 2 2
  spline S140 degree 2 poles (1.0434, 10.8957) (0.9223, 10.7944) (0.6136, 10.6882) (0.3789, 10.6882) knots 0 0 0 1 2 2 2
  line L125 (4.4026, 13.0298) -> (3.8221, 10.7426)
  line L126 (3.8221, 10.7426) -> (3.4665, 10.7426)
  line L127 (3.4665, 10.7426) -> (2.9082, 12.5061)
  line L128 (2.9082, 12.5061) -> (2.3525, 10.7426)
  line L129 (2.3525, 10.7426) -> (1.9993, 10.7426)
  line L130 (1.9993, 10.7426) -> (1.4139, 13.0298)
  line L131 (1.4139, 13.0298) -> (1.814, 13.0298)
  line L132 (1.814, 13.0298) -> (2.2191, 11.2588)
  line L133 (2.2191, 11.2588) -> (2.76, 13.0298)
  line L134 (2.76, 13.0298) -> (3.0787, 13.0298)
  line L135 (3.0787, 13.0298) -> (3.6344, 11.2588)
  line L136 (3.6344, 11.2588) -> (4.0148, 13.0298)
  line L137 (4.0148, 13.0298) -> (4.4026, 13.0298)
  line L138 (5.1337, 10.7426) -> (4.7484, 10.7426)
  line L139 (4.7484, 10.7426) -> (4.7484, 13.0298)
  line L140 (4.7484, 13.0298) -> (5.1337, 13.0298)
  line L141 (5.1337, 13.0298) -> (5.1337, 10.7426)
  line L142 (5.1609, 13.4102) -> (4.7237, 13.4102)
  line L143 (4.7237, 13.4102) -> (4.7237, 13.8103)
  line L144 (4.7237, 13.8103) -> (5.1609, 13.8103)
  line L145 (5.1609, 13.8103) -> (5.1609, 13.4102)
  spline S141 degree 2 poles (6.391, 10.6981) (6.0773, 10.6981) (5.7241, 11.0562) (5.7241, 11.444) knots 0 0 0 1 2 2 2
  line L146 (5.7241, 11.444) -> (5.7241, 12.7112)
  line L147 (5.7241, 12.7112) -> (5.4647, 12.7112)
  line L148 (5.4647, 12.7112) -> (5.4647, 13.0298)
  line L149 (5.4647, 13.0298) -> (5.7241, 13.0298)
  line L150 (5.7241, 13.0298) -> (5.7241, 13.6868)
  line L151 (5.7241, 13.6868) -> (6.1094, 13.6868)
  line L152 (6.1094, 13.6868) -> (6.1094, 13.0298)
  line L153 (6.1094, 13.0298) -> (6.8183, 13.0298)
  line L154 (6.8183, 13.0298) -> (6.8183, 12.7112)
  line L155 (6.8183, 12.7112) -> (6.1094, 12.7112)
  line L156 (6.1094, 12.7112) -> (6.1094, 11.6219)
  spline S142 degree 2 poles (6.1094, 11.6219) (6.1094, 11.449) (6.1217, 11.2588) (6.1637, 11.1773) knots 0 0 0 1 2 2 2
  spline S143 degree 2 poles (6.1637, 11.1773) (6.1983, 11.1056) (6.3539, 11.034) (6.4873, 11.034) knots 0 0 0 1 2 2 2
  spline S144 degree 2 poles (6.4873, 11.034) (6.5812, 11.034) (6.7565, 11.0908) (6.796, 11.1081) knots 0 0 0 1 2 2 2
  line L157 (6.796, 11.1081) -> (6.8183, 11.1081)
  line L158 (6.8183, 11.1081) -> (6.8183, 10.7623)
  spline S145 degree 2 poles (6.8183, 10.7623) (6.7096, 10.7327) (6.4873, 10.6981) (6.391, 10.6981) knots 0 0 0 1 2 2 2
  spline S146 degree 2 poles (8.0113, 10.6907) (7.7742, 10.6907) (7.3814, 10.8364) (7.2407, 10.9846) knots 0 0 0 1 2 2 2
  spline S147 degree 2 poles (7.2407, 10.9846) (7.0999, 11.1303) (6.9442, 11.5799) (6.9442, 11.8812) knots 0 0 0 1 2 2 2
  spline S148 degree 2 poles (6.9442, 11.8812) (6.9442, 12.1826) (7.1048, 12.6222) (7.2407, 12.7704) knots 0 0 0 1 2 2 2
  spline S149 degree 2 poles (7.2407, 12.7704) (7.3765, 12.9211) (7.7791, 13.0817) (8.0113, 13.0817) knots 0 0 0 1 2 2 2
  spline S150 degree 2 poles (8.0113, 13.0817) (8.199, 13.0817) (8.5498, 12.9754) (8.6856, 12.9063) knots 0 0 0 1 2 2 2
  line L159 (8.6856, 12.9063) -> (8.6856, 12.474)
  line L160 (8.6856, 12.474) -> (8.6634, 12.474)
  spline S151 degree 2 poles (8.6634, 12.474) (8.6214, 12.5086) (8.4929, 12.5975) (8.4016, 12.6445) knots 0 0 0 1 2 2 2
  spline S152 degree 2 poles (8.4016, 12.6445) (8.32, 12.684) (8.1027, 12.7457) (8.0039, 12.7457) knots 0 0 0 1 2 2 2
  spline S153 degree 2 poles (8.0039, 12.7457) (7.705, 12.7457) (7.3419, 12.2937) (7.3419, 11.8812) knots 0 0 0 1 2 2 2
  spline S154 degree 2 poles (7.3419, 11.8812) (7.3419, 11.4786) (7.6927, 11.0266) (8.0039, 11.0266) knots 0 0 0 1 2 2 2
  spline S155 degree 2 poles (8.0039, 11.0266) (8.1916, 11.0266) (8.5325, 11.1822) (8.6634, 11.3032) knots 0 0 0 1 2 2 2
  line L161 (8.6634, 11.3032) -> (8.6856, 11.3032)
  line L162 (8.6856, 11.3032) -> (8.6856, 10.871)
  spline S156 degree 2 poles (8.6856, 10.871) (8.6288, 10.8438) (8.4559, 10.7673) (8.3867, 10.75) knots 0 0 0 1 2 2 2
  spline S157 degree 2 poles (8.3867, 10.75) (8.2879, 10.7203) (8.1323, 10.6907) (8.0113, 10.6907) knots 0 0 0 1 2 2 2
  line L163 (10.8321, 10.7426) -> (10.4467, 10.7426)
  line L164 (10.4467, 10.7426) -> (10.4467, 12.0467)
  spline S158 degree 2 poles (10.4467, 12.0467) (10.4467, 12.2048) (10.4171, 12.4765) (10.3726, 12.558) knots 0 0 0 1 2 2 2
  spline S159 degree 2 poles (10.3726, 12.558) (10.3257, 12.6445) (10.1577, 12.7284) (10.0145, 12.7284) knots 0 0 0 1 2 2 2
  spline S160 degree 2 poles (10.0145, 12.7284) (9.8712, 12.7284) (9.5674, 12.5753) (9.4217, 12.4518) knots 0 0 0 1 2 2 2
  line L165 (9.4217, 12.4518) -> (9.4217, 10.7426)
  line L166 (9.4217, 10.7426) -> (9.0364, 10.7426)
  line L167 (9.0364, 10.7426) -> (9.0364, 13.9264)
  line L168 (9.0364, 13.9264) -> (9.4217, 13.9264)
  line L169 (9.4217, 13.9264) -> (9.4217, 12.7754)
  spline S161 degree 2 poles (9.4217, 12.7754) (9.5946, 12.931) (9.928, 13.094) (10.1157, 13.094) knots 0 0 0 1 2 2 2
  spline S162 degree 2 poles (10.1157, 13.094) (10.4517, 13.094) (10.8321, 12.6494) (10.8321, 12.227) knots 0 0 0 1 2 2 2
  line L170 (10.8321, 12.227) -> (10.8321, 10.7426)
  line L171 (-17.3175, -12.7417) -> (-17.3175, -10.0543)
  line L172 (-17.3175, -10.0543) -> (-18.3401, -10.0543)
  line L173 (-18.3401, -10.0543) -> (-18.3401, -9.6937)
  line L174 (-18.3401, -9.6937) -> (-15.8899, -9.6937)
  line L175 (-15.8899, -9.6937) -> (-15.8899, -10.0543)
  line L176 (-15.8899, -10.0543) -> (-16.9125, -10.0543)
  line L177 (-16.9125, -10.0543) -> (-16.9125, -12.7417)
  line L178 (-16.9125, -12.7417) -> (-17.3175, -12.7417)
  line L179 (-15.218, -12.7417) -> (-15.6034, -12.7417)
  line L180 (-15.6034, -12.7417) -> (-15.6034, -10.4545)
  line L181 (-15.6034, -10.4545) -> (-15.218, -10.4545)
  line L182 (-15.218, -10.4545) -> (-15.218, -12.7417)
  line L183 (-15.1909, -10.0741) -> (-15.6281, -10.0741)
  line L184 (-15.6281, -10.0741) -> (-15.6281, -9.6739)
  line L185 (-15.6281, -9.6739) -> (-15.1909, -9.6739)
  line L186 (-15.1909, -9.6739) -> (-15.1909, -10.0741)
  line L187 (-14.2597, -12.7417) -> (-14.645, -12.7417)
  line L188 (-14.645, -12.7417) -> (-14.645, -9.5579)
  line L189 (-14.645, -9.5579) -> (-14.2597, -9.5579)
  line L190 (-14.2597, -9.5579) -> (-14.2597, -12.7417)
  spline S163 degree 2 poles (-11.2067, -11.9488) (-11.2067, -12.349) (-11.6958, -12.7837) (-12.1083, -12.7837) knots 0 0 0 1 2 2 2
  spline S164 degree 2 poles (-12.1083, -12.7837) (-12.2071, -12.7837) (-12.5356, -12.7491) (-12.6467, -12.7244) knots 0 0 0 1 2 2 2
  line L191 (-12.6467, -12.7244) -> (-12.6467, -12.3342)
  line L192 (-12.6467, -12.3342) -> (-12.6245, -12.3342)
  spline S165 degree 2 poles (-12.6245, -12.3342) (-12.5405, -12.3638) (-12.2911, -12.433) (-12.1626, -12.433) knots 0 0 0 1 2 2 2
  spline S166 degree 2 poles (-12.1626, -12.433) (-11.9749, -12.433) (-11.7501, -12.3465) (-11.6983, -12.2675) knots 0 0 0 1 2 2 2
  spline S167 degree 2 poles (-11.6983, -12.2675) (-11.6414, -12.186) (-11.6118, -11.9488) (-11.6118, -11.7932) knots 0 0 0 1 2 2 2
  line L193 (-11.6118, -11.7932) -> (-11.6118, -10.0173)
  line L194 (-11.6118, -10.0173) -> (-12.2565, -10.0173)
  line L195 (-12.2565, -10.0173) -> (-12.2565, -9.6937)
  line L196 (-12.2565, -9.6937) -> (-11.2067, -9.6937)
  line L197 (-11.2067, -9.6937) -> (-11.2067, -11.9488)
  spline S168 degree 2 poles (-9.3641, -12.4996) (-9.411, -12.5342) (-9.5691, -12.6577) (-9.6432, -12.6948) knots 0 0 0 1 2 2 2
  spline S169 degree 2 poles (-9.6432, -12.6948) (-9.7445, -12.7491) (-9.9347, -12.8059) (-10.1076, -12.8059) knots 0 0 0 1 2 2 2
  spline S170 degree 2 poles (-10.1076, -12.8059) (-10.2484, -12.8059) (-10.5028, -12.6997) (-10.5991, -12.6034) knots 0 0 0 1 2 2 2
  spline S171 degree 2 poles (-10.5991, -12.6034) (-10.6905, -12.5095) (-10.8016, -12.2329) (-10.8016, -12.0797) knots 0 0 0 1 2 2 2
  spline S172 degree 2 poles (-10.8016, -12.0797) (-10.8016, -11.8426) (-10.6016, -11.5067) (-10.3842, -11.4104) knots 0 0 0 1 2 2 2
  spline S173 degree 2 poles (-10.3842, -11.4104) (-10.1915, -11.3215) (-9.6679, -11.2548) (-9.3641, -11.2375) knots 0 0 0 1 2 2 2
  line L198 (-9.3641, -11.2375) -> (-9.3641, -11.1634)
  spline S174 degree 2 poles (-9.3641, -11.1634) (-9.3641, -11.03) (-9.4456, -10.8645) (-9.5197, -10.8176) knots 0 0 0 1 2 2 2
  spline S175 degree 2 poles (-9.5197, -10.8176) (-9.5938, -10.7706) (-9.8062, -10.741) (-9.9198, -10.741) knots 0 0 0 1 2 2 2
  spline S176 degree 2 poles (-9.9198, -10.741) (-10.0532, -10.741) (-10.4138, -10.82) (-10.5942, -10.8966) knots 0 0 0 1 2 2 2
  line L199 (-10.5942, -10.8966) -> (-10.6164, -10.8966)
  line L200 (-10.6164, -10.8966) -> (-10.6164, -10.5039)
  spline S177 degree 2 poles (-10.6164, -10.5039) (-10.5102, -10.4742) (-10.1125, -10.4001) (-9.9174, -10.4001) knots 0 0 0 1 2 2 2
  spline S178 degree 2 poles (-9.9174, -10.4001) (-9.6803, -10.4001) (-9.3567, -10.4742) (-9.2282, -10.5706) knots 0 0 0 1 2 2 2
  spline S179 degree 2 poles (-9.2282, -10.5706) (-9.1023, -10.6644) (-8.9788, -10.9633) (-8.9788, -11.1782) knots 0 0 0 1 2 2 2
  line L201 (-8.9788, -11.1782) -> (-8.9788, -12.7417)
  line L202 (-8.9788, -12.7417) -> (-9.3641, -12.7417)
  line L203 (-9.3641, -12.7417) -> (-9.3641, -12.4996)
  line L204 (-9.3641, -12.1785) -> (-9.3641, -11.5438)
  spline S180 degree 2 poles (-9.3641, -11.5438) (-9.5024, -11.5561) (-9.9198, -11.5981) (-10.0508, -11.6376) knots 0 0 0 1 2 2 2
  spline S181 degree 2 poles (-10.0508, -11.6376) (-10.2039, -11.6845) (-10.404, -11.8797) (-10.404, -12.0526) knots 0 0 0 1 2 2 2
  spline S182 degree 2 poles (-10.404, -12.0526) (-10.404, -12.2502) (-10.1817, -12.4502) (-9.9692, -12.4502) knots 0 0 0 1 2 2 2
  spline S183 degree 2 poles (-9.9692, -12.4502) (-9.7889, -12.4502) (-9.4925, -12.2946) (-9.3641, -12.1785) knots 0 0 0 1 2 2 2
  line L205 (-6.6421, -12.7417) -> (-7.0275, -12.7417)
  line L206 (-7.0275, -12.7417) -> (-7.0275, -11.4375)
  spline S184 degree 2 poles (-7.0275, -11.4375) (-7.0275, -11.2795) (-7.0571, -11.0078) (-7.1016, -10.9262) knots 0 0 0 1 2 2 2
  spline S185 degree 2 poles (-7.1016, -10.9262) (-7.1485, -10.8398) (-7.3164, -10.7558) (-7.4597, -10.7558) knots 0 0 0 1 2 2 2
  spline S186 degree 2 poles (-7.4597, -10.7558) (-7.603, -10.7558) (-7.9068, -10.909) (-8.0525, -11.0325) knots 0 0 0 1 2 2 2
  line L207 (-8.0525, -11.0325) -> (-8.0525, -12.7417)
  line L208 (-8.0525, -12.7417) -> (-8.4378, -12.7417)
  line L209 (-8.4378, -12.7417) -> (-8.4378, -10.4545)
  line L210 (-8.4378, -10.4545) -> (-8.0525, -10.4545)
  line L211 (-8.0525, -10.4545) -> (-8.0525, -10.7089)
  spline S187 degree 2 poles (-8.0525, -10.7089) (-7.8796, -10.5533) (-7.5462, -10.3903) (-7.3584, -10.3903) knots 0 0 0 1 2 2 2
  spline S188 degree 2 poles (-7.3584, -10.3903) (-7.0225, -10.3903) (-6.6421, -10.8349) (-6.6421, -11.2572) knots 0 0 0 1 2 2 2
  line L212 (-6.6421, -11.2572) -> (-6.6421, -12.7417)
  line L213 (-2.5493, -12.7417) -> (-2.9544, -12.7417)
  line L214 (-2.9544, -12.7417) -> (-2.9544, -11.2498)
  line L215 (-2.9544, -11.2498) -> (-4.3574, -11.2498)
  line L216 (-4.3574, -11.2498) -> (-4.3574, -12.7417)
  line L217 (-4.3574, -12.7417) -> (-4.7625, -12.7417)
  line L218 (-4.7625, -12.7417) -> (-4.7625, -9.6937)
  line L219 (-4.7625, -9.6937) -> (-4.3574, -9.6937)
  line L220 (-4.3574, -9.6937) -> (-4.3574, -10.8892)
  line L221 (-4.3574, -10.8892) -> (-2.9544, -10.8892)
  line L222 (-2.9544, -10.8892) -> (-2.9544, -9.6937)
  line L223 (-2.9544, -9.6937) -> (-2.5493, -9.6937)
  line L224 (-2.5493, -9.6937) -> (-2.5493, -12.7417)
  spline S189 degree 2 poles (-0.9685, -12.7936) (-1.5169, -12.7936) (-2.1195, -12.1785) (-2.1195, -11.6104) knots 0 0 0 1 2 2 2
  spline S190 degree 2 poles (-2.1195, -11.6104) (-2.1195, -11.0522) (-1.5341, -10.3903) (-1.0624, -10.3903) knots 0 0 0 1 2 2 2
  spline S191 degree 2 poles (-1.0624, -10.3903) (-0.8499, -10.3903) (-0.5214, -10.5138) (-0.4004, -10.6447) knots 0 0 0 1 2 2 2
  spline S192 degree 2 poles (-0.4004, -10.6447) (-0.2769, -10.7756) (-0.146, -11.1535) (-0.146, -11.4277) knots 0 0 0 1 2 2 2
  line L225 (-0.146, -11.4277) -> (-0.146, -11.6376)
  line L226 (-0.146, -11.6376) -> (-1.7293, -11.6376)
  spline S193 degree 2 poles (-1.7293, -11.6376) (-1.7293, -12.0353) (-1.3291, -12.4577) (-0.9734, -12.4577) knots 0 0 0 1 2 2 2
  spline S194 degree 2 poles (-0.9734, -12.4577) (-0.8475, -12.4577) (-0.6029, -12.4008) (-0.5041, -12.3564) knots 0 0 0 1 2 2 2
  spline S195 degree 2 poles (-0.5041, -12.3564) (-0.4004, -12.307) (-0.2571, -12.2205) (-0.2102, -12.181) knots 0 0 0 1 2 2 2
  line L227 (-0.2102, -12.181) -> (-0.188, -12.181)
  line L228 (-0.188, -12.181) -> (-0.188, -12.6009)
  spline S196 degree 2 poles (-0.188, -12.6009) (-0.2547, -12.6281) (-0.4572, -12.7071) (-0.5363, -12.7294) knots 0 0 0 1 2 2 2
  spline S197 degree 2 poles (-0.5363, -12.7294) (-0.6474, -12.7615) (-0.8302, -12.7936) (-0.9685, -12.7936) knots 0 0 0 1 2 2 2
  spline S198 degree 2 poles (-0.5214, -11.3437) (-0.5264, -11.1881) (-0.5906, -10.9608) (-0.6523, -10.8843) knots 0 0 0 1 2 2 2
  spline S199 degree 2 poles (-0.6523, -10.8843) (-0.719, -10.7978) (-0.929, -10.7064) (-1.0846, -10.7064) knots 0 0 0 1 2 2 2
  spline S200 degree 2 poles (-1.0846, -10.7064) (-1.2377, -10.7064) (-1.4526, -10.7978) (-1.5416, -10.8867) knots 0 0 0 1 2 2 2
  spline S201 degree 2 poles (-1.5416, -10.8867) (-1.628, -10.9781) (-1.7169, -11.1979) (-1.7293, -11.3437) knots 0 0 0 1 2 2 2
  line L229 (-1.7293, -11.3437) -> (-0.5214, -11.3437)
  line L230 (0.637, -12.7417) -> (0.2517, -12.7417)
  line L231 (0.2517, -12.7417) -> (0.2517, -9.5579)
  line L232 (0.2517, -9.5579) -> (0.637, -9.5579)
  line L233 (0.637, -9.5579) -> (0.637, -12.7417)
  line L234 (1.5954, -12.7417) -> (1.21, -12.7417)
  line L235 (1.21, -12.7417) -> (1.21, -9.5579)
  line L236 (1.21, -9.5579) -> (1.5954, -9.5579)
  line L237 (1.5954, -9.5579) -> (1.5954, -12.7417)
  spline S202 degree 2 poles (4.0777, -11.561) (4.0777, -12.1217) (3.5343, -12.8059) (3.1243, -12.8059) knots 0 0 0 1 2 2 2
  spline S203 degree 2 poles (3.1243, -12.8059) (2.9391, -12.8059) (2.6748, -12.7145) (2.5463, -12.6355) knots 0 0 0 1 2 2 2
  line L238 (2.5463, -12.6355) -> (2.5216, -12.7417)
  line L239 (2.5216, -12.7417) -> (2.161, -12.7417)
  line L240 (2.161, -12.7417) -> (2.161, -9.5579)
  line L241 (2.161, -9.5579) -> (2.5463, -9.5579)
  line L242 (2.5463, -9.5579) -> (2.5463, -10.6941)
  spline S204 degree 2 poles (2.5463, -10.6941) (2.6921, -10.5632) (3.0304, -10.3903) (3.2453, -10.3903) knots 0 0 0 1 2 2 2
  spline S205 degree 2 poles (3.2453, -10.3903) (3.6331, -10.3903) (4.0777, -11.0102) (4.0777, -11.561) knots 0 0 0 1 2 2 2
  spline S206 degree 2 poles (3.6801, -11.5907) (3.6801, -11.1807) (3.4306, -10.7558) (3.154, -10.7558) knots 0 0 0 1 2 2 2
  spline S207 degree 2 poles (3.154, -10.7558) (2.9983, -10.7558) (2.6772, -10.904) (2.5463, -11.0176) knots 0 0 0 1 2 2 2
  line L243 (2.5463, -11.0176) -> (2.5463, -12.3292)
  spline S208 degree 2 poles (2.5463, -12.3292) (2.6921, -12.4008) (2.9168, -12.4601) (3.0502, -12.4601) knots 0 0 0 1 2 2 2
  spline S209 degree 2 poles (3.0502, -12.4601) (3.3441, -12.4601) (3.6801, -12.0427) (3.6801, -11.5907) knots 0 0 0 1 2 2 2
  spline S210 degree 2 poles (6.3576, -11.5981) (6.3576, -12.1761) (5.8018, -12.8059) (5.3374, -12.8059) knots 0 0 0 1 2 2 2
  spline S211 degree 2 poles (5.3374, -12.8059) (4.8607, -12.8059) (4.3149, -12.1563) (4.3149, -11.5981) knots 0 0 0 1 2 2 2
  spline S212 degree 2 poles (4.3149, -11.5981) (4.3149, -11.025) (4.878, -10.3903) (5.3374, -10.3903) knots 0 0 0 1 2 2 2
  spline S213 degree 2 poles (5.3374, -10.3903) (5.8018, -10.3903) (6.3576, -11.0226) (6.3576, -11.5981) knots 0 0 0 1 2 2 2
  spline S214 degree 2 poles (5.9599, -11.5981) (5.9599, -11.1535) (5.6363, -10.7212) (5.3374, -10.7212) knots 0 0 0 1 2 2 2
  spline S215 degree 2 poles (5.3374, -10.7212) (5.0386, -10.7212) (4.7125, -11.1535) (4.7125, -11.5981) knots 0 0 0 1 2 2 2
  spline S216 degree 2 poles (4.7125, -11.5981) (4.7125, -12.0303) (5.0386, -12.4749) (5.3374, -12.4749) knots 0 0 0 1 2 2 2
  spline S217 degree 2 poles (5.3374, -12.4749) (5.6338, -12.4749) (5.9599, -12.0378) (5.9599, -11.5981) knots 0 0 0 1 2 2 2
  line L244 (8.5485, -10.4545) -> (7.3184, -13.584)
  line L245 (7.3184, -13.584) -> (6.9059, -13.584)
  line L246 (6.9059, -13.584) -> (7.3159, -12.6306)
  line L247 (7.3159, -12.6306) -> (6.486, -10.4545)
  line L248 (6.486, -10.4545) -> (6.901, -10.4545)
  line L249 (6.901, -10.4545) -> (7.5259, -12.1489)
  line L250 (7.5259, -12.1489) -> (8.1483, -10.4545)
  line L251 (8.1483, -10.4545) -> (8.5485, -10.4545)
  line L252 (-16.8557, -14.9468) -> (-16.8754, -14.9468)
  spline S218 degree 2 poles (-16.8754, -14.9468) (-16.9273, -14.9271) (-17.1199, -14.8925) (-17.1965, -14.8925) knots 0 0 0 1 2 2 2
  spline S219 degree 2 poles (-17.1965, -14.8925) (-17.4386, -14.8925) (-17.6461, -15.1098) (-17.6461, -15.3964) knots 0 0 0 1 2 2 2
  line L253 (-17.6461, -15.3964) -> (-17.6461, -15.4729)
  line L254 (-17.6461, -15.4729) -> (-17.0088, -15.4729)
  line L255 (-17.0088, -15.4729) -> (-17.0088, -15.7916)
  line L256 (-17.0088, -15.7916) -> (-17.6337, -15.7916)
  line L257 (-17.6337, -15.7916) -> (-17.6337, -17.7602)
  line L258 (-17.6337, -17.7602) -> (-18.019, -17.7602)
  line L259 (-18.019, -17.7602) -> (-18.019, -15.7916)
  line L260 (-18.019, -15.7916) -> (-18.2784, -15.7916)
  line L261 (-18.2784, -15.7916) -> (-18.2784, -15.4729)
  line L262 (-18.2784, -15.4729) -> (-18.019, -15.4729)
  line L263 (-18.019, -15.4729) -> (-18.019, -15.3964)
  spline S220 degree 2 poles (-18.019, -15.3964) (-18.019, -14.9863) (-17.6214, -14.5566) (-17.2509, -14.5566) knots 0 0 0 1 2 2 2
  spline S221 degree 2 poles (-17.2509, -14.5566) (-17.1446, -14.5566) (-16.9396, -14.5788) (-16.8557, -14.5936) knots 0 0 0 1 2 2 2
  line L264 (-16.8557, -14.5936) -> (-16.8557, -14.9468)
  line L265 (-15.512, -15.8854) -> (-15.5317, -15.8854)
  spline S222 degree 2 poles (-15.5317, -15.8854) (-15.5762, -15.8731) (-15.6725, -15.8681) (-15.7392, -15.8681) knots 0 0 0 1 2 2 2
  spline S223 degree 2 poles (-15.7392, -15.8681) (-15.8948, -15.8681) (-16.2011, -16.004) (-16.3394, -16.1374) knots 0 0 0 1 2 2 2
  line L266 (-16.3394, -16.1374) -> (-16.3394, -17.7602)
  line L267 (-16.3394, -17.7602) -> (-16.7247, -17.7602)
  line L268 (-16.7247, -17.7602) -> (-16.7247, -15.4729)
  line L269 (-16.7247, -15.4729) -> (-16.3394, -15.4729)
  line L270 (-16.3394, -15.4729) -> (-16.3394, -15.8138)
  spline S224 degree 2 poles (-16.3394, -15.8138) (-16.1295, -15.6261) (-15.8158, -15.4729) (-15.6676, -15.4729) knots 0 0 0 1 2 2 2
  spline S225 degree 2 poles (-15.6676, -15.4729) (-15.6083, -15.4729) (-15.549, -15.4779) (-15.512, -15.4853) knots 0 0 0 1 2 2 2
  line L271 (-15.512, -15.4853) -> (-15.512, -15.8854)
  spline S226 degree 2 poles (-13.9386, -17.5181) (-13.9855, -17.5527) (-14.1436, -17.6762) (-14.2177, -17.7132) knots 0 0 0 1 2 2 2
  spline S227 degree 2 poles (-14.2177, -17.7132) (-14.3189, -17.7676) (-14.5091, -17.8244) (-14.682, -17.8244) knots 0 0 0 1 2 2 2
  spline S228 degree 2 poles (-14.682, -17.8244) (-14.8228, -17.8244) (-15.0772, -17.7182) (-15.1736, -17.6218) knots 0 0 0 1 2 2 2
  spline S229 degree 2 poles (-15.1736, -17.6218) (-15.265, -17.528) (-15.3761, -17.2513) (-15.3761, -17.0982) knots 0 0 0 1 2 2 2
  spline S230 degree 2 poles (-15.3761, -17.0982) (-15.3761, -16.8611) (-15.176, -16.5252) (-14.9587, -16.4288) knots 0 0 0 1 2 2 2
  spline S231 degree 2 poles (-14.9587, -16.4288) (-14.766, -16.3399) (-14.2424, -16.2732) (-13.9386, -16.2559) knots 0 0 0 1 2 2 2
  line L272 (-13.9386, -16.2559) -> (-13.9386, -16.1818)
  spline S232 degree 2 poles (-13.9386, -16.1818) (-13.9386, -16.0484) (-14.0201, -15.8829) (-14.0942, -15.836) knots 0 0 0 1 2 2 2
  spline S233 degree 2 poles (-14.0942, -15.836) (-14.1683, -15.7891) (-14.3807, -15.7594) (-14.4943, -15.7594) knots 0 0 0 1 2 2 2
  spline S234 degree 2 poles (-14.4943, -15.7594) (-14.6277, -15.7594) (-14.9883, -15.8385) (-15.1686, -15.9151) knots 0 0 0 1 2 2 2
  line L273 (-15.1686, -15.9151) -> (-15.1909, -15.9151)
  line L274 (-15.1909, -15.9151) -> (-15.1909, -15.5223)
  spline S235 degree 2 poles (-15.1909, -15.5223) (-15.0846, -15.4927) (-14.687, -15.4186) (-14.4918, -15.4186) knots 0 0 0 1 2 2 2
  spline S236 degree 2 poles (-14.4918, -15.4186) (-14.2547, -15.4186) (-13.9312, -15.4927) (-13.8027, -15.589) knots 0 0 0 1 2 2 2
  spline S237 degree 2 poles (-13.8027, -15.589) (-13.6767, -15.6829) (-13.5532, -15.9817) (-13.5532, -16.1966) knots 0 0 0 1 2 2 2
  line L275 (-13.5532, -16.1966) -> (-13.5532, -17.7602)
  line L276 (-13.5532, -17.7602) -> (-13.9386, -17.7602)
  line L277 (-13.9386, -17.7602) -> (-13.9386, -17.5181)
  line L278 (-13.9386, -17.197) -> (-13.9386, -16.5622)
  spline S238 degree 2 poles (-13.9386, -16.5622) (-14.0769, -16.5746) (-14.4943, -16.6165) (-14.6252, -16.6561) knots 0 0 0 1 2 2 2
  spline S239 degree 2 poles (-14.6252, -16.6561) (-14.7784, -16.703) (-14.9784, -16.8981) (-14.9784, -17.071) knots 0 0 0 1 2 2 2
  spline S240 degree 2 poles (-14.9784, -17.071) (-14.9784, -17.2686) (-14.7561, -17.4687) (-14.5437, -17.4687) knots 0 0 0 1 2 2 2
  spline S241 degree 2 poles (-14.5437, -17.4687) (-14.3634, -17.4687) (-14.067, -17.3131) (-13.9386, -17.197) knots 0 0 0 1 2 2 2
  line L279 (-11.6736, -17.7602) -> (-11.6736, -14.7122)
  line L280 (-11.6736, -14.7122) -> (-9.7667, -14.7122)
  line L281 (-9.7667, -14.7122) -> (-9.7667, -15.0728)
  line L282 (-9.7667, -15.0728) -> (-11.2685, -15.0728)
  line L283 (-11.2685, -15.0728) -> (-11.2685, -15.9076)
  line L284 (-11.2685, -15.9076) -> (-9.868, -15.9076)
  line L285 (-9.868, -15.9076) -> (-9.868, -16.2683)
  line L286 (-9.868, -16.2683) -> (-11.2685, -16.2683)
  line L287 (-11.2685, -16.2683) -> (-11.2685, -17.3995)
  line L288 (-11.2685, -17.3995) -> (-9.7667, -17.3995)
  line L289 (-9.7667, -17.3995) -> (-9.7667, -17.7602)
  line L290 (-9.7667, -17.7602) -> (-11.6736, -17.7602)
  spline S242 degree 2 poles (-8.4724, -17.8145) (-8.8034, -17.8145) (-9.2678, -17.6762) (-9.4728, -17.5774) knots 0 0 0 1 2 2 2
  line L291 (-9.4728, -17.5774) -> (-9.4728, -17.0686)
  line L292 (-9.4728, -17.0686) -> (-9.4431, -17.0686)
  spline S243 degree 2 poles (-9.4431, -17.0686) (-9.2431, -17.2563) (-8.7367, -17.4638) (-8.5021, -17.4638) knots 0 0 0 1 2 2 2
  spline S244 degree 2 poles (-8.5021, -17.4638) (-8.1661, -17.4638) (-7.8228, -17.1846) (-7.8228, -16.9549) knots 0 0 0 1 2 2 2
  spline S245 degree 2 poles (-7.8228, -16.9549) (-7.8228, -16.7722) (-8.0031, -16.5449) (-8.1982, -16.4881) knots 0 0 0 1 2 2 2
  spline S246 degree 2 poles (-8.1982, -16.4881) (-8.339, -16.4486) (-8.5737, -16.3942) (-8.7491, -16.3498) knots 0 0 0 1 2 2 2
  spline S247 degree 2 poles (-8.7491, -16.3498) (-8.9071, -16.3078) (-9.1566, -16.1818) (-9.2529, -16.0806) knots 0 0 0 1 2 2 2
  spline S248 degree 2 poles (-9.2529, -16.0806) (-9.3468, -15.9793) (-9.4505, -15.7076) (-9.4505, -15.5297) knots 0 0 0 1 2 2 2
  spline S249 degree 2 poles (-9.4505, -15.5297) (-9.4505, -15.1592) (-8.8726, -14.6578) (-8.4255, -14.6578) knots 0 0 0 1 2 2 2
  spline S250 degree 2 poles (-8.4255, -14.6578) (-8.1686, -14.6578) (-7.7141, -14.7591) (-7.519, -14.8554) knots 0 0 0 1 2 2 2
  line L293 (-7.519, -14.8554) -> (-7.519, -15.3395)
  line L294 (-7.519, -15.3395) -> (-7.5486, -15.3395)
  spline S251 degree 2 poles (-7.5486, -15.3395) (-7.6944, -15.2062) (-8.1488, -15.0086) (-8.3983, -15.0086) knots 0 0 0 1 2 2 2
  spline S252 degree 2 poles (-8.3983, -15.0086) (-8.6799, -15.0086) (-9.0282, -15.2729) (-9.0282, -15.4877) knots 0 0 0 1 2 2 2
  spline S253 degree 2 poles (-9.0282, -15.4877) (-9.0282, -15.6804) (-8.8232, -15.9101) (-8.6305, -15.962) knots 0 0 0 1 2 2 2
  spline S254 degree 2 poles (-8.6305, -15.962) (-8.5021, -15.9966) (-8.1291, -16.0855) (-8.0056, -16.1225) knots 0 0 0 1 2 2 2
  spline S255 degree 2 poles (-8.0056, -16.1225) (-7.6919, -16.2189) (-7.4004, -16.6067) (-7.4004, -16.8907) knots 0 0 0 1 2 2 2
  spline S256 degree 2 poles (-7.4004, -16.8907) (-7.4004, -17.071) (-7.5462, -17.4168) (-7.6771, -17.5379) knots 0 0 0 1 2 2 2
  spline S257 degree 2 poles (-7.6771, -17.5379) (-7.8228, -17.6712) (-8.1933, -17.8145) (-8.4724, -17.8145) knots 0 0 0 1 2 2 2
  spline S258 degree 2 poles (-4.5846, -16.2386) (-4.5846, -16.6561) (-4.923, -17.3279) (-5.2071, -17.5156) knots 0 0 0 1 2 2 2